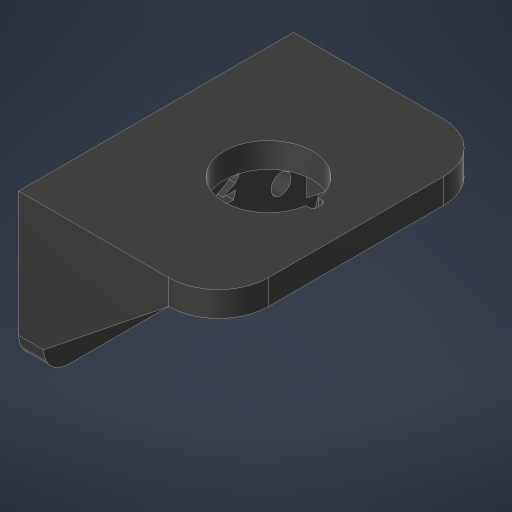
# Autodesk Inventor part: rsl mount
Saved by Autodesk Inventor 2023.4 (Build 274418000, 418)
## iProperties
Created: 2025-02-28
Part Number: rsl mount
Material: ABS Plastic
Document SubType Name: Modeling
Designer: brand
Density: 1.06 g/cm^3
Appearance: Smooth - Black
Author: brand
Autodesk Inventor part; units mm, degrees
ref_plane "YZ Plane" through (0, 0, 0) normal (1, 0, 0) x (0, 1, 0)
ref_plane "XZ Plane" through (0, 0, 0) normal (0, 1, 0) x (-1, 0, 0)
ref_plane "XY Plane" through (0, 0, 0) normal (0, 0, 1) x (1, 0, 0)
sketch "Sketch1" plane through (0, 0, 0) normal (0, 0, 1) x (1, 0, 0)
  line L0 (0, 0) -> (50.8, 0)
  line L1 (50.8, 0) -> (50.8, -6.35)
  line L2 (50.8, -6.35) -> (6.35, -6.35)
  line L3 (6.35, -6.35) -> (6.35, -38.1)
  line L4 (6.35, -38.1) -> (0, -38.1)
  line L5 (0, -38.1) -> (0, 0)
  dimension "d0" = 50.8
  dimension "d1" = 38.1
  dimension "d2" = 6.35
  dimension "d3" = 6.35
  constraints: 12 end point, 5 perpendicular, 1 horizontal
  measures "d0" distance of L0.start L0.end
  measures "d1" distance of L4.end L0.start
  measures "d2" distance of L0.end L1.end
  measures "d3" distance of L3.end L4.end
extrude "Extrusion1" add sketch "Sketch1" along normal mid plane 69.85
sketch "Sketch2" plane through (0, 0, 34.925) normal (0, 1, 0) x (1, 0, 0)
  line L0 (0, 69.85) -> (0, 0) construction
  line L1 (50.8, 0) -> (0, 0) construction
  line L2 (50.8, 69.85) -> (50.8, 0) construction
  line L3 (0, 69.85) -> (50.8, 69.85) construction
  circle A0 centre (28.575, 34.925) radius 11.2522
  line L4 (0, 0) -> (0, 69.85) construction
  line L5 (6.35, 69.85) -> (6.35, 0) construction
  line L6 (6.35, 69.85) -> (6.35, 0) construction
  line L7 (6.35, 69.85) -> (6.35, 0) construction
  line L8 (6.35, 69.85) -> (50.8, 69.85) construction
  line L9 (41.525, 36.525) -> (41.525, 33.325)
  line L10 (41.525, 36.525) -> (39.7129, 36.525)
  line L11 (41.525, 33.325) -> (39.7129, 33.325)
  point P0 (0, 34.925)
  point P1 (0, 34.925)
  point P2 (28.575, 69.85)
  point P3 (41.525, 34.925)
  dimension "d6" = 22.5044
  dimension "d16" = 3.2
  dimension "d17" = 12.95
  constraints: 8 end point, 3 midpoint, 2 horizontal, 2 horizontal alignment, 2 point on circle, 1 centre point, 1 perpendicular, 1 vertical, 1 vertical alignment
  measures "d6" diameter of A0
  measures "d16" distance of L9.start L9.end
  measures "d17" distance from line of L9 A0.centre
sketch "Sketch3" plane through (0, -38.1, 34.925) normal (-1, 0, 0) x (0, 0, 1)
  line L0 (0, 0) -> (-69.85, 0) construction
  line L1 (0, 38.1) -> (0, 0) construction
  line L2 (-69.85, 38.1) -> (0, 38.1) construction
  line L3 (-69.85, 0) -> (-69.85, 38.1) construction
  line L4 (-9.525, 25.4) -> (-60.325, 25.4) construction
  line L5 (-60.325, 25.4) -> (-60.325, 12.7) construction
  line L6 (-60.325, 12.7) -> (-9.525, 12.7) construction
  line L7 (-9.525, 12.7) -> (-9.525, 25.4) construction
  line L8 (-9.525, 25.4) -> (-60.325, 12.7) construction
  line L9 (-60.325, 25.4) -> (-9.525, 12.7) construction
  point P0 (-34.925, 38.1)
  point P1 (-34.925, 19.05)
  point P2 (-34.925, 38.1)
  point P3 (0, 19.05)
  dimension "d7" = 50.8
  dimension "d8" = 12.7
  constraints: 12 end point, 4 coincident, 4 midpoint, 2 parallel, 1 horizontal, 1 horizontal alignment, 1 perpendicular, 1 vertical alignment
  measures "d7" distance of L5.end L6.end
  measures "d8" distance of L4.end L5.end
hole "Hole1" at (0, -12.7, -25.4) at (0, -25.4, -25.4) at (0, -25.4, 25.4) at (0, -12.7, 25.4) direction (1, 0, 0) diameter 5.1054 end through all clearance for "Flat Head Machine Screw (82)" size "#10" standard "Ansi Unified Screw Threads"
extrude "Extrusion2" cut sketch "Sketch2" against normal through all
fillet "Fillet1" radius 0.8 2 edges at (41.525, -3.175, -1.6) (41.525, -3.175, 1.6)
fillet "Fillet2" radius 12.7 2 edges at (50.8, -3.175, -34.925) (50.8, -3.175, 34.925)
fillet "Fillet3" radius 6.35 2 edges at (3.175, -38.1, -34.925) (3.175, -38.1, 34.925)
sketch "Sketch5" plane through (0, 0, -34.925) normal (0, 0, -1) x (-1, 0, 0)
  line L0 (0, -31.75) -> (-6.35, -31.75) construction
  line L1 (0, -31.75) -> (0, 0) construction
  line L2 (0, 0) -> (-38.1, 0) construction
  line L3 (-38.1, -6.35) -> (-38.1, 0) construction
  line L4 (-38.1, -6.35) -> (-6.35, -6.35) construction
  line L5 (-6.35, -6.35) -> (-6.35, -31.75) construction
  line L6 (-38.1, -6.35) -> (-6.35, -31.75)
  line L7 (-6.35, -6.35) -> (-6.35, -31.75)
  line L8 (-6.35, -27.9527) -> (-6.35, -22.8473) construction
  line L9 (-6.35, -6.35) -> (-38.1, -6.35)
  line L10 (-17.3228, -6.35) -> (-39.7129, -6.35) construction
  constraints: 6 end point, 2 collinear
extrude "Extrusion3" add sketch "Sketch5" against normal blind 3
mirror "Mirror1" about plane through (0, 0, 0) normal (0, 0, 1) of "Extrusion3"
fillet "Fillet4" radius 6.35 2 edges at (22.225, -6.35, 31.925) (22.225, -6.35, -31.925)
sketch "Sketch6" plane through (6.35, -38.1, 28.575) normal (1, 0, 0) x (0, 0, -1)
  line L0 (13.6613, 22.86) -> (43.4887, 22.86) construction
  line L1 (43.4887, 22.86) -> (43.4887, 15.24) construction
  line L2 (43.4887, 15.24) -> (13.6613, 15.24) construction
  line L3 (13.6613, 15.24) -> (13.6613, 22.86) construction
  line L4 (50.8, 38.1) -> (6.35, 38.1) construction
  circle A0 centre (3.175, 25.4) radius 2.5527 construction
  circle A1 centre (3.175, 12.7) radius 2.5527 construction
  line L5 (3.175, 25.4) -> (3.175, 12.7) construction
  line L6 (13.5219, 15.2158) -> (19.8931, 15.2279)
  line L7 (19.8931, 15.2279) -> (20.4266, 17.1071)
  line L8 (20.4266, 17.1071) -> (17.2197, 17.1071)
  spline S0 degree 2 poles (17.2197, 17.1071) (17.6805, 17.4951) (19.881, 18.3498) (20.3356, 18.6893) knots 0 0 0 1 2 2 2
  spline S1 degree 2 poles (20.3356, 18.6893) (21.1237, 19.3076) (21.3298, 20.2836) knots 0 0 0 1 1 1
  line L9 (21.3298, 20.2836) -> (18.5352, 20.2836)
  spline S2 degree 2 poles (18.5352, 20.2836) (18.5473, 20.2594) (18.5473, 20.2291) knots 0 0 0 1 1 1
  spline S3 degree 2 poles (18.5473, 20.2291) (18.5473, 19.9199) (17.3955, 19.3743) knots 0 0 0 1 1 1
  spline S4 degree 2 poles (17.3955, 19.3743) (15.6921, 18.5802) (14.995, 17.9922) knots 0 0 0 1 1 1
  spline S5 degree 2 poles (14.995, 17.9922) (13.631, 16.8646) (13.5219, 15.2158) knots 0 0 0 1 1 1
  spline S6 degree 2 poles (21.4207, 21.0232) (21.4207, 21.7082) (21.2025, 22.0962) knots 0 0 0 1 1 1
  spline S7 degree 2 poles (21.2025, 22.0962) (20.7782, 22.86) (20.1477, 22.86) knots 0 0 0 1 1 1
  line L10 (20.1477, 22.86) -> (17.438, 22.86)
  spline S8 degree 2 poles (17.438, 22.86) (16.7105, 22.86) (15.3466, 21.7446) (15.1041, 21.0232) knots 0 0 0 1 2 2 2
  line L11 (15.1041, 21.0232) -> (21.4207, 21.0232)
  line L12 (20.8145, 15.2158) -> (27.1858, 15.2279)
  line L13 (27.1858, 15.2279) -> (27.7192, 17.1071)
  line L14 (27.7192, 17.1071) -> (24.5124, 17.1071)
  spline S9 degree 2 poles (24.5124, 17.1071) (24.9731, 17.4951) (27.1736, 18.3498) (27.6283, 18.6893) knots 0 0 0 1 2 2 2
  spline S10 degree 2 poles (27.6283, 18.6893) (28.4163, 19.3076) (28.6225, 20.2836) knots 0 0 0 1 1 1
  line L15 (28.6225, 20.2836) -> (25.8279, 20.2836)
  spline S11 degree 2 poles (25.8279, 20.2836) (25.84, 20.2594) (25.84, 20.2291) knots 0 0 0 1 1 1
  spline S12 degree 2 poles (25.84, 20.2291) (25.84, 19.9199) (24.6882, 19.3743) knots 0 0 0 1 1 1
  spline S13 degree 2 poles (24.6882, 19.3743) (22.9847, 18.5802) (22.2876, 17.9922) knots 0 0 0 1 1 1
  spline S14 degree 2 poles (22.2876, 17.9922) (20.9237, 16.8646) (20.8145, 15.2158) knots 0 0 0 1 1 1
  spline S15 degree 2 poles (28.7134, 21.0232) (28.7134, 21.7082) (28.4952, 22.0962) knots 0 0 0 1 1 1
  spline S16 degree 2 poles (28.4952, 22.0962) (28.0708, 22.86) (27.4404, 22.86) knots 0 0 0 1 1 1
  line L16 (27.4404, 22.86) -> (24.7306, 22.86)
  spline S17 degree 2 poles (24.7306, 22.86) (24.0032, 22.86) (22.6392, 21.7446) (22.3967, 21.0232) knots 0 0 0 1 2 2 2
  line L17 (22.3967, 21.0232) -> (28.7134, 21.0232)
  spline S18 degree 2 poles (31.9626, 18.3135) (32.4234, 18.3135) (32.6113, 18.271) knots 0 0 0 1 1 1
  spline S19 degree 2 poles (32.6113, 18.271) (33.0114, 18.168) (33.0114, 17.8467) knots 0 0 0 1 1 1
  spline S20 degree 2 poles (33.0114, 17.8467) (33.0114, 17.5375) (32.5567, 17.0526) (32.2354, 17.0283) knots 0 0 0 1 2 2 2
  spline S21 degree 2 poles (32.2354, 17.0283) (32.0051, 17.0101) (31.8717, 17.0101) knots 0 0 0 1 1 1
  spline S22 degree 2 poles (31.8717, 17.0101) (31.2291, 17.0101) (31.2291, 17.4163) knots 0 0 0 1 1 1
  spline S23 degree 2 poles (31.2291, 17.4163) (31.2291, 17.4951) (31.2413, 17.5739) knots 0 0 0 1 1 1
  line L18 (31.2413, 17.5739) -> (28.7619, 17.5739)
  spline S24 degree 2 poles (28.7619, 17.5739) (28.6528, 16.8768) (28.7073, 16.6282) knots 0 0 0 1 1 1
  spline S25 degree 2 poles (28.7073, 16.6282) (28.9922, 15.2158) (30.5684, 15.2158) knots 0 0 0 1 1 1
  line L19 (30.5684, 15.2158) -> (32.7447, 15.2158)
  spline S26 degree 2 poles (32.7447, 15.2158) (33.2417, 15.2946) (33.8176, 15.6583) knots 0 0 0 1 1 1
  spline S27 degree 2 poles (33.8176, 15.6583) (34.3269, 15.9796) (34.5572, 16.2766) knots 0 0 0 1 1 1
  spline S28 degree 2 poles (34.5572, 16.2766) (35.1331, 17.0222) (35.2543, 17.974) knots 0 0 0 1 1 1
  spline S29 degree 2 poles (35.2543, 17.974) (35.2665, 18.1013) (35.2665, 18.2225) knots 0 0 0 1 1 1
  spline S30 degree 2 poles (35.2665, 18.2225) (35.2665, 18.8894) (34.9149, 19.3198) knots 0 0 0 1 1 1
  spline S31 degree 2 poles (34.9149, 19.3198) (34.4905, 19.8714) (33.3751, 20.2836) (32.5689, 20.2836) knots 0 0 0 1 2 2 2
  line L20 (32.5689, 20.2836) -> (29.5621, 20.2836)
  line L21 (29.5621, 20.2836) -> (28.9922, 18.3135)
  line L22 (28.9922, 18.3135) -> (31.9626, 18.3135)
  line L23 (35.6544, 21.0232) -> (29.0529, 21.0232)
  line L24 (29.0529, 21.0232) -> (30.2228, 22.86)
  line L25 (30.2228, 22.86) -> (36.2061, 22.86)
  line L26 (36.2061, 22.86) -> (35.6544, 21.0232)
  line L27 (35.5453, 15.2158) -> (41.9165, 15.2279)
  line L28 (41.9165, 15.2279) -> (42.45, 17.1071)
  line L29 (42.45, 17.1071) -> (39.2432, 17.1071)
  spline S32 degree 2 poles (39.2432, 17.1071) (39.7039, 17.4951) (41.9044, 18.3498) (42.3591, 18.6893) knots 0 0 0 1 2 2 2
  spline S33 degree 2 poles (42.3591, 18.6893) (43.1471, 19.3076) (43.3532, 20.2836) knots 0 0 0 1 1 1
  line L30 (43.3532, 20.2836) -> (40.5586, 20.2836)
  spline S34 degree 2 poles (40.5586, 20.2836) (40.5708, 20.2594) (40.5708, 20.2291) knots 0 0 0 1 1 1
  spline S35 degree 2 poles (40.5708, 20.2291) (40.5708, 19.9199) (39.419, 19.3743) knots 0 0 0 1 1 1
  spline S36 degree 2 poles (39.419, 19.3743) (37.7155, 18.5802) (37.0184, 17.9922) knots 0 0 0 1 1 1
  spline S37 degree 2 poles (37.0184, 17.9922) (35.6544, 16.8646) (35.5453, 15.2158) knots 0 0 0 1 1 1
  spline S38 degree 2 poles (43.4442, 21.0232) (43.4442, 21.7082) (43.2259, 22.0962) knots 0 0 0 1 1 1
  spline S39 degree 2 poles (43.2259, 22.0962) (42.8016, 22.86) (42.1711, 22.86) knots 0 0 0 1 1 1
  line L31 (42.1711, 22.86) -> (39.4614, 22.86)
  spline S40 degree 2 poles (39.4614, 22.86) (38.734, 22.86) (37.37, 21.7446) (37.1275, 21.0232) knots 0 0 0 1 2 2 2
  line L32 (37.1275, 21.0232) -> (43.4442, 21.0232)
  point P0 (28.575, 38.1)
  point P1 (28.575, 22.86)
  point P2 (28.575, 38.1)
  point P3 (13.6613, 19.05)
  point P4 (3.175, 19.05)
  dimension "d0" = 50.8
  dimension "d1" = 38.1
  dimension "d2" = 6.35
  dimension "d3" = 6.35
  dimension "d29" = 7.62
  dimension "d30" = 29.8274
  constraints: 4 midpoint, 2 end point, 1 horizontal alignment, 1 vertical, 1 vertical alignment, 2 other
  measures "d29" distance of L2.end L0.start
  measures "d30" distance of L0.start L0.end
extrude "Extrusion4" cut sketch "Sketch6" against normal through all
body "Solid1"
